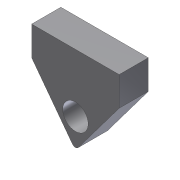
# Autodesk Inventor part: LauncherBearingBlockRepresentation
Saved by Autodesk Inventor 2012 (Build 160160000, 160)
## iProperties
Created: 2013-01-12
Part Number: LauncherBearingBlockRepresentation
Material: Default
Document SubType Name: Modeling
Designer: JesseK
Density: 1 g/cm^3
Mass: 88.3645 g
Surface Area: 151.174 cm^2
Volume: 88.3645 cm^3
Author: JesseK
Autodesk Inventor part; units mm, degrees
ref_plane "YZ Plane" through (0, 0, 0) normal (1, 0, 0) x (0, 1, 0)
ref_plane "XZ Plane" through (0, 0, 0) normal (0, 1, 0) x (-1, 0, 0)
ref_plane "XY Plane" through (0, 0, 0) normal (0, 0, 1) x (1, 0, 0)
sketch "Sketch1" plane through (0, 0, 0) normal (0, 0, 1) x (1, 0, 0)
  line L0 (0, 0) -> (0, -25.4)
  line L1 (0, -25.4) -> (38.1, -76.2)
  line L2 (38.1, -76.2) -> (76.2, -25.4)
  line L3 (76.2, -25.4) -> (76.2, 0)
  line L4 (76.2, 0) -> (0, 0)
  circle A0 centre (38.1, -50.8) radius 11.1125
  line L5 (0, 0) -> (38.1, -50.8) construction
  line L6 (38.1, -50.8) -> (76.2, 0) construction
  dimension "d0" = 76.2
  dimension "d1" = 25.4
  dimension "d2" = 50.8
  dimension "d3" = 22.225
  dimension "d4" = 50.8
  constraints: 14 end point, 2 equal length, 2 vertical, 1 centre point, 1 horizontal
  measures "d0" distance of L3.end L0.start
  measures "d1" distance from line of L2.end L4
  measures "d2" vertical distance of L0.end L1.end
  measures "d3" diameter of A0
  measures "d4" distance from line of L4 L5.end
extrude "Extrusion1" add sketch "Sketch1" along normal blind 25.4
fillet "Fillet1" radius 3.175 1 edges at (38.1, -76.2, 12.7)
body "Solid1"
